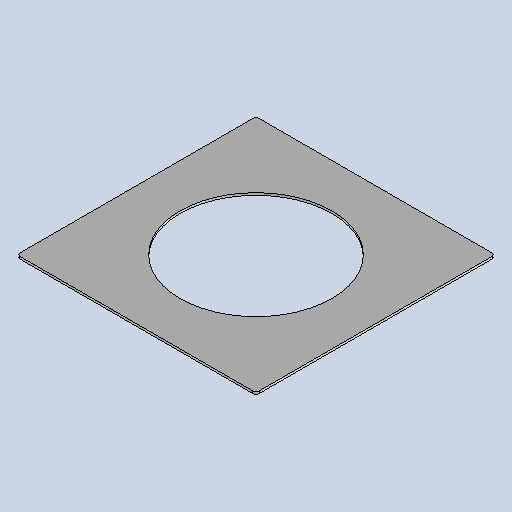
# Autodesk Inventor part: TKS 3003 BOTTOM DS reduce flange
Saved by Autodesk Inventor 2025.1 (Build 291241020, 241B)
## iProperties
Created: 2024-12-09
Part Number: TKS 3003 BOTTOM DS reduce flange
Material: Stainless Steel
Document SubType Name: Sheet Metal
Designer: user
Mass: 3269.02 g
Surface Area: 1007.63 cm^2
Volume: 408.627 cm^3
Density: 8 g/cm^3
Flat Pattern Width: 31.5 cm
Flat Pattern Length: 31.5 cm
Flat Pattern Area: 992.25 cm^2
Sheet Metal Rule: AISI304 3mm Die 32
Sheet Metal Width: 315.000 mm
Sheet Metal Length: 315.000 mm
Sheet Metal Area: 99225.000 mm^2
Appearance: Default
Author: user
Autodesk Inventor part; units mm, degrees
ref_plane "YZ Plane" through (0, 0, 0) normal (1, 0, 0) x (0, 1, 0)
ref_plane "XZ Plane" through (0, 0, 0) normal (0, 1, 0) x (-1, 0, 0)
ref_plane "XY Plane" through (0, 0, 0) normal (0, 0, 1) x (1, 0, 0)
sketch "Sketch1" plane through (0, 0, 0) normal (0, 0, 1) x (1, 0, 0)
  circle A0 centre (0, 0) radius 100
  circle A1 centre (0, 0) radius 157.5
  line L0 (157.5, 157.5) -> (-157.5, 157.5)
  line L1 (-157.5, 157.5) -> (-157.5, -157.5)
  line L2 (-157.5, -157.5) -> (157.5, -157.5)
  line L3 (157.5, -157.5) -> (157.5, 157.5)
  line L4 (157.5, 157.5) -> (-157.5, -157.5) construction
  line L5 (-157.5, 157.5) -> (157.5, -157.5) construction
  point P0 (157.5, 0)
  point P1 (0, -157.5)
  point P2 (0, 157.5)
  point P3 (-157.5, 0)
  dimension "d22" = 200
  dimension "d23" = 315
  measures "d22" diameter of A0
  measures "d23" diameter of A1
extrude "Plate1" add sketch "Sketch1" along normal blind 3
fillet "Corner Round1" radius 4 4 edges at (157.5, -157.5, 1.5) (157.5, 157.5, 1.5) (-157.5, 157.5, 1.5) (-157.5, -157.5, 1.5)
equation "\"d2\" = Thickness"
equation "\"BendReliefWidth\" = Thickness"
equation "\"BendReliefDepth\" = 0.5 * Thickness"
equation "\"CornerReliefSize\" = 4 * Thickness"
equation "\"MinimumRemnant\" = 2 * Thickness"
equation "\"TransitionRadius\" = BendRadius"
equation "\"JacobiRadiusSize\" = BendRadius"
equation "\"GapSize\" = Thickness"
equation "\"Thickness\" = 3"
equation "\"BendRadius\" = 5"
body "Solid1"
